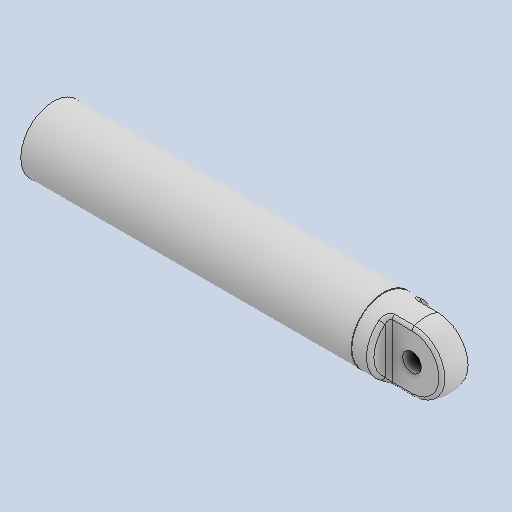
# Autodesk Inventor part: ANT-38-Shaft
Saved by Autodesk Inventor 2025.2 (Build 292293000, 293)
## iProperties
Created: 2026-01-25
Part Number: ANT-38-Shaft
Material: Generic
Document SubType Name: Modeling
Designer: LattePanda
Density: 1 g/cm^3
Appearance: Default
Author: LattePanda
Autodesk Inventor part; units mm, degrees
sketch "Body" plane through (0, 0, 0) normal (0, 1, 0) x (-1, 0, 0)
  circle A0 centre (0, 0) radius 5
  circle A1 centre (0, 0) radius 17.5
  line L0 (0, -17.5) -> (200, -17.5)
  line L1 (200, -17.5) -> (200, 17.5)
  line L2 (200, 17.5) -> (0, 17.5)
  line L3 (0, 17.5) -> (0, -17.5)
  line L4 (243.5, 0) -> (-61, 0) construction
  line L5 (0, -24.5) -> (0, 24.5) construction
  line L6 (-17.5, 0) -> (200, 0)
  point P0 (0, 0)
  dimension "d0" = 10
  dimension "d1" = 35
  dimension "d2" = 35
  dimension "d3" = 200
  constraints: 10 end point, 3 point on line, 2 centre point, 2 coincident, 2 midpoint, 2 parallel, 2 point on circle, 1 horizontal, 1 perpendicular
  measures "d0" diameter of A0
  measures "d1" diameter of A1
  measures "d2" distance of L2.end L0.start
  measures "d3" distance between parallel lines of L1 L3
revolve "BodyFeature" add sketch "Body" angle 360 about axis through (17.5, 0, 0) along (-1, 0, 0) picked at (13.1453, -1.6689) picked at (1.7623, -2.8047) picked at (-1.6689, -13.1453) picked at (-0.3709, -3.2915) contours L6 A1 L3 A0 | A0 L3 L6 | L3 A1 L6 A0 | A0 L6 L3 | L6 L1 L0 A1
ref_plane "Work Plane1" through (0, 0, -7.5) normal (0, 0, 1) x (1, 0, 0)
ref_plane "Work Plane2" through (0, 0, 7.5) normal (0, 0, 1) x (1, 0, 0)
sketch "Sketch2" plane through (0, 0, -7.5) normal (0, 0, 1) x (1, 0, 0)
  arc A0 (0, -17.5) -> (0, 17.5) centre (0, 0) ccw projected
  arc A1 (0, -17.5) -> (0, 17.5) centre (0, 0) ccw
  line L0 (0, -17.5) -> (0, -17.5) construction
  line L1 (0, 17.5) -> (0, -17.5) construction
  line L2 (0, -17.5) -> (-12.5, -17.5)
  line L3 (-12.5, -17.5) -> (-12.5, 17.5)
  line L4 (-12.5, 17.5) -> (0, 17.5)
  line L5 (-12.5, 17.5) -> (-12.5, -17.5)
  dimension "d8" = 12.5
  constraints: 10 end point, 2 point on circle, 1 centre point, 1 collinear, 1 concentric, 1 horizontal, 1 parallel, 1 perpendicular, 1 point on line
  measures "d8" distance between parallel lines of L1 L3
extrude "Extrusion1" cut sketch "Sketch2" against normal through all
mirror "Mirror1" about plane through (0, 0, 0) normal (0, 0, 1) of "Extrusion1"
sketch "Sketch3" plane through (0, 0, -7.5) normal (0, 0, -1) x (-1, 0, 0)
  circle A0 centre (0, 0) radius 5
  dimension "d11" = 10
  constraints: 1 centre point, 1 coincident
  measures "d11" diameter of A0
extrude "Extrusion2" cut sketch "Sketch3" against normal through all
fillet "Fillet2" radius 2 2 edges at (-12.5, 0, -7.5) (-12.5, 0, 7.5)
ref_plane "Work Plane5" through (-22.5, 0, 0) normal (1, 0, 0) x (0, 0, -1)
sketch "Sketch6" plane through (-22.5, 0, 0) normal (1, 0, 0) x (0, 0, -1)
  circle A0 centre (0, 0) radius 17.5 projected
  circle A1 centre (0, 0) radius 17.25
  point P0 (0, 0)
  dimension "d28" = 0.25
  constraints: 1 centre point
  measures "d28" radial gap between concentric circles of A0 A1
extrude "Extrusion5" cut sketch "Sketch6" along normal mid plane 0.25
fillet "Fillet3" radius 2 12 edges at (-12.5, 0, 17.5) (15.8114, 0, 7.5) (-5.25, -15.8114, 7.5) (-5.25, 15.8114, 7.5) (-5.25, 15.8114, -7.5) (-11.8919, 15.5314, -8.0638) (-12.5, -8.3666, -15.3704) (-12.5, 8.3666, -15.3704) (-11.8919, -15.5314, -8.0638) (-5.25, -15.8114, -7.5) (11.1803, 11.1803, -7.5) (11.1803, -11.1803, -7.5)
body "Solid1"
